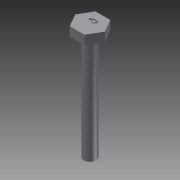
# Autodesk Inventor part: .2'' diameter 2.5 inch bolts for wheel
Saved by Autodesk Inventor 2011 SP1 (Build 150282100, 282)
## iProperties
Created: 2013-01-18
Part Number: .2'' diameter 2.5 inch bolts for wheel
Document SubType Name: Modeling
Designer: wes
Density: 1 g/cm^3
Author: wes
Autodesk Inventor part; units mm, degrees
ref_plane "YZ Plane" through (0, 0, 0) normal (1, 0, 0) x (0, 1, 0)
ref_plane "XZ Plane" through (0, 0, 0) normal (0, 1, 0) x (-1, 0, 0)
ref_plane "XY Plane" through (0, 0, 0) normal (0, 0, 1) x (1, 0, 0)
sketch "Sketch1" plane through (0, 0, 0) normal (0, 0, 1) x (1, 0, 0)
  line L0 (-85.3474, 52.3284) -> (-82.8074, 52.3284)
  line L1 (-82.8074, 52.3284) -> (-82.8074, 7.8784)
  line L2 (-82.8074, 7.8784) -> (-85.3474, 7.8784)
  line L3 (-85.3474, 7.8784) -> (-85.3474, 52.3284)
  point P0 (0, 0)
  dimension "d0" = 2.54
  dimension "d1" = 44.45
  constraints: 8 end point, 2 parallel, 1 horizontal, 1 perpendicular
  measures "d0" distance of L0.start L0.end
  measures "d1" distance of L0.end L1.end
revolve "Revolution1" add sketch "Sketch1" angle 360 about axis through (-85.3474, 7.8784, 0) along (0, 1, 0)
sketch "Sketch2" plane through (-85.3474, 52.3284, 0) normal (0, 1, 0) x (1, 0, 0)
  circle A0 centre (0, 0) radius 2.54 projected
  line L0 (6.1828, 0) -> (3.0914, -5.3544)
  line L1 (3.0914, -5.3544) -> (-3.0914, -5.3544)
  line L2 (-3.0914, -5.3544) -> (-6.1828, 0)
  line L3 (-6.1828, 0) -> (-3.0914, 5.3544)
  line L4 (-3.0914, 5.3544) -> (3.0914, 5.3544)
  line L5 (3.0914, 5.3544) -> (6.1828, 0)
  point P0 (85.3474, 0)
  constraints: 12 end point, 1 coincident, 13 other
extrude "Extrusion1" add sketch "Sketch2" along normal blind 3.81 contours A0 | L0 L1 L2 L3 L4 L5
sketch "Sketch3" plane through (-85.3474, 56.1384, 0) normal (0, 1, 0) x (1, 0, 0)
  line L0 (-3.0914, 5.3544) -> (3.0914, 5.3544) projected
  ellipse E0 centre (0, 1.4435) end of major axis (0, 0.4462) minor radius 1.8269
  spline S0 degree 5 poles (-0.9642, 1.0834) (-0.9417, 0.9678) (-0.7135, 0.7937) (0.1443, 0.7781) (1.4903, 0.7931) (0.5526, 1.6401) (0.1051, 0.6276) (-0.4914, 1.4752) (-0.8935, 1.3263) (-0.9814, 1.1718) (-0.9642, 1.0834) knots 0 0 0 0 0 0 0.230424 0.370543 0.547944 0.706233 0.823711 1 1 1 1 1 1
  circle A0 centre (-0.9642, 1.8591) radius 0.1959
  circle A1 centre (0.6426, 1.8591) radius 0.277
  point P0 (85.3474, 0)
  point P1 (0.9196, 1.0834)
  point P2 (0.6426, 1.2496)
  point P3 (0, 1.0834)
  point P4 (-0.7703, 1.305)
  constraints: 2 centre point, 1 horizontal, 8 other
extrude "Extrusion2" cut sketch "Sketch3" against normal blind 0.508
body "Solid1"
